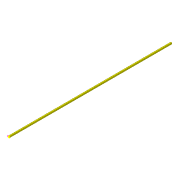
# Autodesk Inventor part: thin rod
Saved by Autodesk Inventor 2016 (Build 200138000, 138)
## iProperties
Created: 2016-07-27
Part Number: thin rod
Material: Polyethylene, High Density
Document SubType Name: Modeling
Designer: dingx
Mass: 18.4112 g
Surface Area: 244.306 cm^2
Volume: 19.3395 cm^3
Density: 0.952 g/cm^3
Appearance: Smooth - Yellow
Author: dingx
Autodesk Inventor part; units mm, degrees
ref_plane "YZ Plane" through (0, 0, 0) normal (1, 0, 0) x (0, 1, 0)
ref_plane "XZ Plane" through (0, 0, 0) normal (0, 1, 0) x (-1, 0, 0)
ref_plane "XY Plane" through (0, 0, 0) normal (0, 0, 1) x (1, 0, 0)
sketch "Sketch1" plane through (0, 0, 0) normal (0, 0, 1) x (1, 0, 0)
  arc A0 (-1.5748, -2.3876) -> (-1.5748, 2.3876) centre (-1.5748, 0) ccw
  line L0 (-1.5748, 2.3876) -> (-3.1623, 2.3876)
  line L1 (-1.5748, -2.3876) -> (-3.1623, -2.3876)
  line L2 (2.286, -2.54) -> (2.286, 2.54)
  line L3 (2.286, 2.54) -> (3.0412, 2.54)
  line L4 (2.286, -2.54) -> (3.0412, -2.54)
  arc A1 (-3.1623, -2.3876) -> (3.0412, -2.54) centre (0, 0) ccw
  arc A2 (3.0412, 2.54) -> (-3.1623, 2.3876) centre (0, 0) ccw
  point P0 (2.286, 0)
  dimension "d2" = 1.5748
  dimension "d3" = 5.08
  dimension "d4" = 2.286
  dimension "d5" = 3.9624
  dimension "d13" = 3.9624
  dimension "d14" = 0.1524
  dimension "d15" = 2.3876
  constraints: 10 end point, 6 point on circle, 3 centre point, 2 horizontal, 2 parallel, 2 tangent, 1 coincident, 1 horizontal alignment, 1 midpoint, 1 vertical
  measures "d2" distance of point (0, 0) A0.centre
  measures "d3" distance of L2.start L2.end
  measures "d4" distance of point (2.286, 0) point (0, 0)
  measures "d5" radius of A2
  measures "d13" radius of A1
  measures "d14" distance between parallel lines of L0 L3
  measures "d15" radius of A0
extrude "Extrusion1" add sketch "Sketch1" along normal blind 787.4
sketch "Sketch2" plane through (0, 0, 787.4) normal (0, 0, 1) x (1, 0, 0)
  arc A0 (-1.5748, -2.3876) -> (-1.5748, 2.3876) centre (-1.5748, 0) ccw projected
  line L0 (-1.5748, -2.3876) -> (-3.1623, -2.3876) projected
  arc A1 (-3.1623, -2.3876) -> (3.0412, -2.54) centre (0, 0) ccw projected
  line L1 (3.0412, -2.54) -> (2.286, -2.54) projected
  line L2 (2.286, -2.54) -> (2.286, 2.54) projected
  line L3 (2.286, 2.54) -> (3.0412, 2.54) projected
  arc A2 (3.0412, 2.54) -> (-3.1623, 2.3876) centre (0, 0) ccw projected
  line L4 (-3.1623, 2.3876) -> (-1.5748, 2.3876) projected
sketch "Sketch3" plane through (0, 0, 787.4) normal (0, 0, 1) x (1, 0, 0)
  arc A0 (-1.5748, -2.3876) -> (-1.5748, 2.3876) centre (-1.5748, 0) ccw projected
  line L0 (-1.5748, -2.3876) -> (-3.1623, -2.3876) projected
  arc A1 (-3.1623, -2.3876) -> (3.0412, -2.54) centre (0, 0) ccw projected
  line L1 (3.0412, -2.54) -> (2.286, -2.54) projected
  line L2 (2.286, -2.54) -> (2.286, 2.54) projected
  line L3 (2.286, 2.54) -> (3.0412, 2.54) projected
  arc A2 (3.0412, 2.54) -> (-3.1623, 2.3876) centre (0, 0) ccw projected
  line L4 (-3.1623, 2.3876) -> (-1.5748, 2.3876) projected
sketch "Sketch4" plane through (0, 0, 787.4) normal (0, 0, 1) x (1, 0, 0)
  arc A0 (-1.5748, -2.3876) -> (-1.5748, 2.3876) centre (-1.5748, 0) ccw projected
  line L0 (-1.5748, -2.3876) -> (-3.1623, -2.3876) projected
  arc A1 (-3.1623, -2.3876) -> (3.0412, -2.54) centre (0, 0) ccw projected
  line L1 (3.0412, -2.54) -> (2.286, -2.54) projected
  line L2 (2.286, -2.54) -> (2.286, 2.54) projected
  line L3 (2.286, 2.54) -> (3.0412, 2.54) projected
  arc A2 (3.0412, 2.54) -> (-3.1623, 2.3876) centre (0, 0) ccw projected
  line L4 (-3.1623, 2.3876) -> (-1.5748, 2.3876) projected
body "Solid1"
